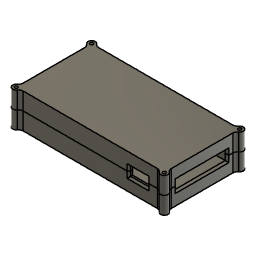
battery_xiaomi-powerbank-20000mAh_box (Autodesk Fusion 360 design; units mm, degrees)
Autodesk Fusion 360 part; units mm, degrees
sketch "Sketch1" plane through (0, 0, 0) normal (0, 1, 0) x (1, 0, 0)
  line L0 (0, 0) -> (155, 0)
  line L1 (155, 0) -> (155, -75)
  line L2 (155, -75) -> (0, -75)
  line L3 (0, -75) -> (0, 0)
  line L4 (159, -79) -> (-4, -79)
  line L5 (-4, -79) -> (-4, 4)
  line L6 (-4, 4) -> (159, 4)
  line L7 (159, 4) -> (159, -79)
  dimension "d5" = 155
  dimension "d6" = 75
  constraint horizontal L0
  constraint vertical L1
  constraint horizontal L2
  constraint vertical L3
  constraint coincident L0.start L3.end
  measures "d5" distance of L0.start L0.end
  measures "d6" distance of L0.start L2.end
extrude "Extrude1" add sketch "Sketch1" along normal blind 30 makes body 1
extrude "Extrude2" add sketch "Sketch1" against normal blind 4 contours L0 L1 L2 L3 | L4 L5 L6 L7 bodies 1
sketch "Sketch3" plane through (0, 30, 0) normal (0, 1, 0) x (-1, 0, 0)
  line L0 (-155, 75) -> (0, 75)
  line L1 (0, 75) -> (0, 0)
  line L2 (0, 0) -> (-155, 0)
  line L3 (-155, 0) -> (-155, 75)
  line L4 (-159, -4) -> (4, -4)
  line L5 (4, -4) -> (4, 79)
  line L6 (4, 79) -> (-159, 79)
  line L7 (-159, 79) -> (-159, -4)
extrude "Extrude3" add sketch "Sketch3" along normal blind 4 contours L0 L1 L2 L3 | L4 L5 L6 L7 bodies 1
sketch "Sketch4" plane through (159, 0, 0) normal (1, 0, 0) x (0, 0, -1)
  line L0 (4, -4) -> (4, 34)
  line L1 (4, 34) -> (-79, 34)
  line L2 (-79, 34) -> (-79, -4)
  line L3 (-79, -4) -> (4, -4)
  line L4 (-67, 8) -> (-8, 8)
  line L5 (-8, 8) -> (-8, 22)
  line L6 (-8, 22) -> (-67, 22)
  line L7 (-67, 22) -> (-67, 8)
  dimension "d14" = -12
extrude "Extrude4" cut sketch "Sketch4" against normal blind 4 contours L4 L5 L6 L7 bodies 1
sketch "Sketch5" plane through (0, 0, 79) normal (0, 0, 1) x (1, 0, 0)
  line L0 (159, -4) -> (159, 34)
  line L1 (159, 34) -> (-4, 34)
  line L2 (-4, 34) -> (-4, -4)
  line L3 (-4, -4) -> (159, -4)
  line L4 (-4, 15) -> (159, 15)
  line L5 (0, 0) -> (155, 0)
  line L6 (155, 0) -> (155, 30)
  line L7 (155, 30) -> (0, 30)
  line L8 (0, 30) -> (0, 0)
  line L9 (155, 15) -> (130, 15)
  line L10 (120, 20) -> (140, 20)
  line L11 (140, 20) -> (140, 10)
  line L12 (140, 10) -> (120, 10)
  line L13 (120, 10) -> (120, 20)
  line L14 (120, 20) -> (140, 10) construction
  line L15 (140, 20) -> (120, 10) construction
  point P0 (130, 15)
  dimension "d18" = 25
  dimension "d19" = 20
  dimension "d20" = 10
  constraint midpoint L2 L4.start
  constraint midpoint L0 L4.end
  constraint midpoint L6 L9.start
  constraint perpendicular L6 L9
  constraint horizontal L10
  constraint perpendicular L10 L11
  constraint parallel L10 L12
  constraint parallel L11 L13
  constraint coincident L14 P0
  constraint coincident L15 P0
  constraint coincident P0 L9.end
  measures "d18" distance of L9.start P0
  measures "d19" distance of L11.end L12.end
  measures "d20" distance of L10.end L11.end
extrude "Extrude5" cut sketch "Sketch5" against normal up to surface (4 mm away) contours L4 L9 L11 L12 L13 | L4 L9 L10 L11 L13 bodies 1
sketch "Sketch6" plane through (0, 34, 0) normal (0, 1, 0) x (-1, 0, 0)
  line L0 (-159, 79) -> (-159, -4)
  line L1 (-159, -4) -> (4, -4)
  line L2 (4, -4) -> (4, 79)
  line L3 (4, 79) -> (-159, 79)
  circle A0 centre (4, -4) radius 4
  circle A1 centre (4, -4) radius 1.25
  line L4 (4, 37.5) -> (-159, 37.5)
  line L5 (-77.5, -4) -> (-77.5, 79)
  circle A2 centre (4, 79) radius 1.25
  circle A3 centre (4, 79) radius 4
  circle A4 centre (-159, -4) radius 1.25
  circle A5 centre (-159, -4) radius 4
  circle A6 centre (-159, 79) radius 1.25
  circle A7 centre (-159, 79) radius 4
  dimension "d23" = 8
  dimension "d24" = 2.5
  constraint coincident L1.end L2.start
  constraint concentric A0 A1
  constraint midpoint L2 L4.start
  constraint midpoint L0 L4.end
  constraint midpoint L1 L5.start
  constraint midpoint L3 L5.end
  constraint symmetric A0 L4 A3
  constraint symmetric A1 L4 A2
  constraint symmetric A0 L5 A5
  constraint symmetric A1 L5 A4
  constraint symmetric L5 A2 A6
  constraint symmetric L5 A3 A7
  measures "d23" diameter of A0
  measures "d24" diameter of A1
extrude "Extrude6" add sketch "Sketch6" against normal up to surface (38 mm away) contours L0 L3 A6 A7 | L0 L1 A4 A5 | L2 L3 A2 A3 | L1 L2 A0 A1 picked at (-160.5423, 76.3396) picked at (-159.7036, -1.0065) picked at (1.6155, 80.9414) picked at (7.0684, -4.1987) bodies 1
extrude "Extrude7" cut sketch "Sketch6" against normal up to surface (38 mm away) contours L0 L3 A6 | L0 L1 A4 | L2 L3 A2 | L1 L2 A1 picked at (-158.9407, 78.1709) picked at (-158.9407, -3.1709) picked at (3.1709, 78.9407) picked at (3.2705, -3.6016) bodies 1
fillet "Fillet1" radius 5 8 edges at (-4, 15, 75) (155, 15, 79) (-4, 15, 0) (159, 15, 0) (0, 15, 79) (0, 15, -4) (159, 15, 75) (155, 15, -4) on bodies 1
chamfer "Chamfer1" distance 2 angle 45 4 edges at (130, 20, 79) (120, 15, 79) (130, 10, 79) (140, 15, 79) on bodies 1
ref_plane "WorkPlane1" through (77.5, 15, 37.5) normal (0, 1, 0) x (1, 0, 0)
split "Split1" by plane through (77.5, 15, 37.5) normal (0, 1, 0) bodies 1 makes body 2 at (52.8278, 34, 23.6667)
copy_body "Body->Comp1" bodies 1 removing the originals makes body 3 in component "bottom"
copy_body "Body->Comp2" bodies 2 removing the originals makes body 4 in component "top"
sketch "Sketch7" plane through (0, 34, 0) normal (0, 1, 0) x (-1, 0, 0)
  arc A0 (-161.2222, -0.6741) -> (-155.6741, -6.2222) centre (-159, -4) ccw
  arc A1 (-151.5167, -4) -> (-155.6741, -6.2222) centre (-151.5167, -9) ccw
  line L0 (-151.5167, -4) -> (-3.4833, -4)
  arc A2 (0.6741, -6.2222) -> (-3.4833, -4) centre (-3.4833, -9) ccw
  arc A3 (0.6741, -6.2222) -> (6.2222, -0.6741) centre (4, -4) ccw
  arc A4 (4, 3.4833) -> (6.2222, -0.6741) centre (9, 3.4833) ccw
  line L1 (4, 3.4833) -> (4, 71.5167)
  arc A5 (6.2222, 75.6741) -> (4, 71.5167) centre (9, 71.5167) ccw
  arc A6 (6.2222, 75.6741) -> (0.6741, 81.2222) centre (4, 79) ccw
  arc A7 (-3.4833, 79) -> (0.6741, 81.2222) centre (-3.4833, 84) ccw
  line L2 (-3.4833, 79) -> (-151.5167, 79)
  arc A8 (-155.6741, 81.2222) -> (-151.5167, 79) centre (-151.5167, 84) ccw
  arc A9 (-155.6741, 81.2222) -> (-161.2222, 75.6741) centre (-159, 79) ccw
  arc A10 (-159, 71.5167) -> (-161.2222, 75.6741) centre (-164, 71.5167) ccw
  line L3 (-159, 71.5167) -> (-159, 3.4833)
  arc A11 (-161.2222, -0.6741) -> (-159, 3.4833) centre (-164, 3.4833) ccw
  circle A12 centre (-159, -4) radius 1.25
  circle A13 centre (4, -4) radius 1.25
  circle A14 centre (4, 79) radius 1.25
  circle A15 centre (-159, 79) radius 1.25
  circle A16 centre (4, -4) radius 1.75
  circle A17 centre (4, 79) radius 1.75
  circle A18 centre (-159, 79) radius 1.75
  circle A19 centre (-159, -4) radius 1.75
  dimension "d33" = 3.5
  dimension "d34" = 3.5
  dimension "d35" = 3.5
  dimension "d36" = 3.5
  constraint concentric A3 A16
  constraint concentric A6 A17
  constraint concentric A9 A18
  constraint concentric A0 A19
  measures "d33" diameter of A16
  measures "d34" diameter of A17
  measures "d35" diameter of A18
  measures "d36" diameter of A19
extrude "Extrude1'" cut sketch "Sketch7" against normal up to surface (19 mm away) contours A16 | A17 | A18 | A19 bodies 4 in component "top"
component "bottom" placed x (1, 0, 0) y (0, 1, 0) z (0, 0, 1) at (0, 0, 0)
component "top" placed x (1, 0, 0) y (0, 1, 0) z (0, 0, 1) at (0, 0, 0)
equation "width = 75 mm"
equation "length = 155 mm"
equation "height = 30 mm"
equation "case_thickness = 4 mm"
equation "d5 = length"
equation "d6 = width"
equation "d7 = -case_thickness"
equation "d8 = height"
equation "d10 = -case_thickness"
equation "d12 = case_thickness"
equation "d14 = -case_thickness - 8 mm"
equation "d15 = -case_thickness"
equation "d17 = -case_thickness"
equation "d32 = height / 2"
